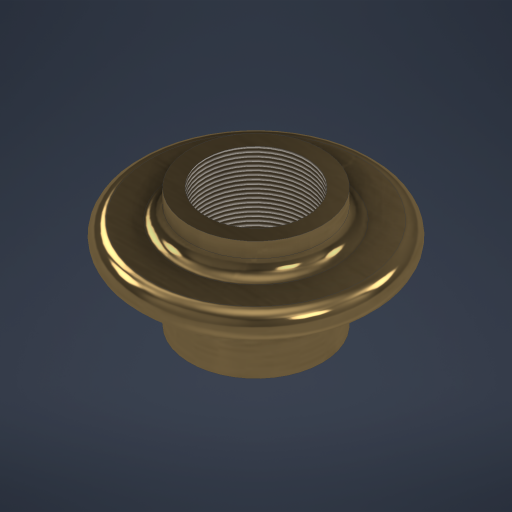
# Autodesk Inventor part: nut
Saved by Autodesk Inventor 2023 (Build 270158000, 158)
## iProperties
Created: 2023-03-09
Part Number: nut
Material: Brass, Soft Yellow, Welded
Document SubType Name: Modeling
Designer: kamraj
Density: 8.5 g/cm^3
Appearance: Brass - Satin 1
Author: kamraj
Autodesk Inventor part; units mm, degrees
ref_plane "YZ Plane" through (0, 0, 0) normal (1, 0, 0) x (0, 1, 0)
ref_plane "XZ Plane" through (0, 0, 0) normal (0, 1, 0) x (-1, 0, 0)
ref_plane "XY Plane" through (0, 0, 0) normal (0, 0, 1) x (1, 0, 0)
sketch "Sketch1" plane through (0, 0, 0) normal (0, 0, 1) x (1, 0, 0)
  line L0 (0, 0) -> (0, 45)
  line L1 (19, 0) -> (19, 45)
  line L2 (19, 45) -> (25, 45)
  line L3 (25, 45) -> (25, 34.25)
  line L4 (25, 34.25) -> (40, 34.25)
  line L5 (40, 24.25) -> (25, 24.25)
  line L6 (25, 24.25) -> (25, 0)
  line L7 (25, 0) -> (19, 0)
  arc A0 (40, 24.25) -> (40, 34.25) centre (40, 29.25) ccw
  point P0 (45, 29.25)
  dimension "d2" = 45
  dimension "d3" = 38
  dimension "d4" = 6
  dimension "d6" = 10
  dimension "d8" = 90
  constraints: 16 end point, 4 perpendicular, 3 point on circle, 2 point on line, 1 centre point, 1 horizontal alignment, 1 parallel, 1 tangent, 1 vertical
  measures "d2" distance of L1.start L1.end
  measures "d3" diameter of L1 L0
  measures "d4" distance of L6.end L1.start
  measures "d6" distance between parallel lines of L5 L4
  measures "d8" diameter of point (45, 29.25) L0
revolve "Revolution1" add sketch "Sketch1" angle 360 about axis through (0, 0, 0) along (0, 1, 0)
fillet "Fillet1" radius 5 2 edges at (-25, 34.25, 0) (-25, 24.25, 0)
thread "Thread1" size "M38x1.5" class "6H" standard "ISO Metric profile" full length
